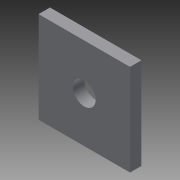
# Autodesk Inventor part: P1-5
Saved by Autodesk Inventor 2014 (Build 180170000, 170)
## iProperties
Created: 2017-02-06
Part Number: P1-5
Material: Generic
Document SubType Name: Modeling
Designer: mschaffel
Density: 1 g/cm^3
Appearance: Default
Author: mschaffel
Autodesk Inventor part; units mm, degrees
ref_plane "YZ Plane" through (0, 0, 0) normal (1, 0, 0) x (0, 1, 0)
ref_plane "XZ Plane" through (0, 0, 0) normal (0, 1, 0) x (-1, 0, 0)
ref_plane "XY Plane" through (0, 0, 0) normal (0, 0, 1) x (1, 0, 0)
sketch "Sketch1" plane through (0, 0, 0) normal (0, 1, 0) x (-1, 0, 0)
  line L0 (0, 0) -> (0, 80)
  line L1 (0, 80) -> (80, 80)
  line L2 (80, 80) -> (80, 0)
  line L3 (80, 0) -> (0, 0)
  circle A0 centre (40, 40) radius 10
  dimension "d0" = 80
  constraints: 8 end point, 2 parallel, 1 centre point, 1 perpendicular, 1 vertical
  measures "d0" distance of L0.start L0.end
extrude "Extrusion1" add sketch "Sketch1" along normal blind 10
body "Solid1"
